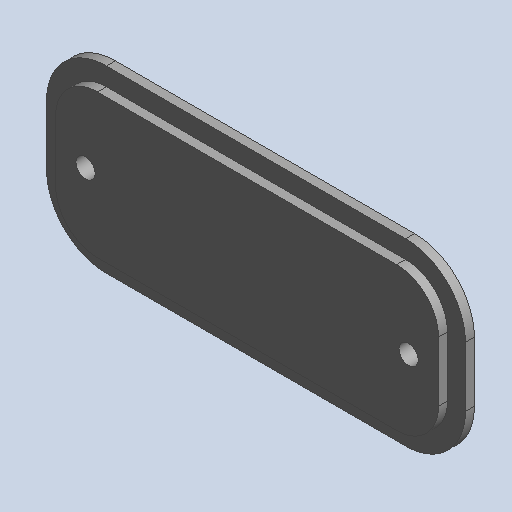
# Autodesk Inventor part: sensor_cover_ultrasonic_2
Saved by Autodesk Inventor 2026 (Build 300175050, 175E)
## iProperties
Part Number: sensor_cover_ultrasonic_2
Material: Generic
Document SubType Name: Modeling
Designer: Kartik
Mass: 5.21389 g
Surface Area: 45.7669 cm^2
Volume: 5.21389 cm^3
Density: 1 g/cm^3
Appearance: Default
Author: Kartik
Autodesk Inventor part; units mm, degrees
ref_plane "YZ Plane" through (0, 0, 0) normal (1, 0, 0) x (0, 1, 0)
ref_plane "XZ Plane" through (0, 0, 0) normal (0, 1, 0) x (-1, 0, 0)
ref_plane "XY Plane" through (0, 0, 0) normal (0, 0, 1) x (1, 0, 0)
sketch "Sketch1" plane through (0, 0, 0) normal (0, 0, 1) x (1, 0, 0)
  line L0 (-35, 15) -> (35, 15)
  line L1 (35, 15) -> (35, -15)
  line L2 (35, -15) -> (-35, -15)
  line L3 (-35, -15) -> (-35, 15)
  point P0 (0, 0)
  dimension "d0" = 70
  dimension "d1" = 30
  dimension "d7" = 35
  dimension "d8" = 15
  constraints: 8 end point, 2 parallel, 1 horizontal, 1 perpendicular
  measures "d0" distance of L0.start L0.end
  measures "d1" distance of L2.end L0.start
  measures "d7" distance from line of L3 point (0, 0)
  measures "d8" distance from line of L0 point (0, 0)
extrude "Extrusion1" add sketch "Sketch1" along normal blind 3
fillet "Fillet1" radius 10 4 edges at (-35, 15, 1.5) (-35, -15, 1.5) (35, -15, 1.5) (35, 15, 1.5)
sketch "Sketch6" plane through (0, 0, 3) normal (0, 0, 1) x (1, 0, 0)
  arc A0 (35, 5) -> (25, 15) centre (25, 5) ccw projected
  line L0 (25, 15) -> (-25, 15) projected
  arc A1 (-25, 15) -> (-35, 5) centre (-25, 5) ccw projected
  line L1 (-35, 5) -> (-35, -5) projected
  arc A2 (-35, -5) -> (-25, -15) centre (-25, -5) ccw projected
  line L2 (-25, -15) -> (25, -15) projected
  arc A3 (25, -15) -> (35, -5) centre (25, -5) ccw projected
  line L3 (35, -5) -> (35, 5) projected
  arc A4 (-25, 12) -> (-32, 5) centre (-25, 5) ccw
  line L4 (-25, 12) -> (25, 12)
  arc A5 (32, 5) -> (25, 12) centre (25, 5) ccw
  line L5 (32, 5) -> (32, -5)
  arc A6 (25, -12) -> (32, -5) centre (25, -5) ccw
  line L6 (25, -12) -> (-25, -12)
  arc A7 (-32, -5) -> (-25, -12) centre (-25, -5) ccw
  line L7 (-32, -5) -> (-32, 5)
  point P0 (0, 0)
  dimension "d43" = 3
  constraints: 8 end point, 8 point on circle, 4 centre point, 7 other
  measures "d43" radial gap between concentric circles of A1 A4
extrude "Extrusion5" cut sketch "Sketch6" against normal blind 1.5
sketch "Sketch7" plane through (0, 0, 3) normal (0, 0, 1) x (1, 0, 0)
  line L0 (-35, -5) -> (-35, 5) projected
  line L1 (35, 5) -> (35, -5) projected
  circle A0 centre (-27, 0) radius 1.6
  circle A1 centre (27, 0) radius 1.6
  point P0 (0, 0)
  point P1 (-35, 0)
  dimension "d46" = 3.2
  dimension "d47" = 8
  dimension "d48" = 3.2
  dimension "d49" = 8
  constraints: 2 centre point, 1 midpoint
  measures "d46" diameter of A0
  measures "d47" distance of point (-35, 0) A0.centre
  measures "d48" diameter of A1
  measures "d49" distance from line of L1 A1.centre
extrude "Extrusion6" cut sketch "Sketch7" against normal through all
equation "\"d7\" = 0.5 * d0"
equation "\"d8\" = 0.5 * d1"
body "Solid1"
